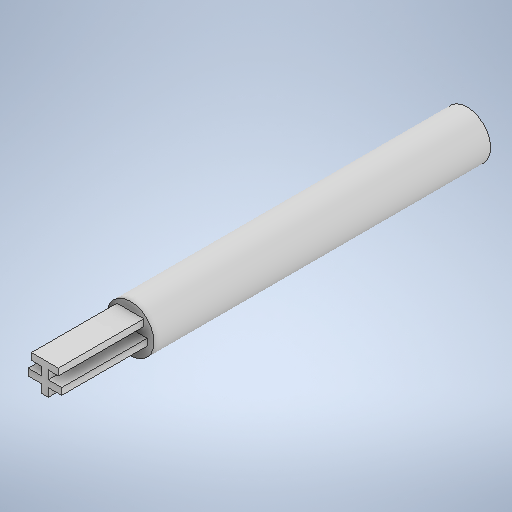
# Autodesk Inventor part: rod attachment(wheelside)
Saved by Autodesk Inventor 2025 (Build 290162000, 162)
## iProperties
Created: 2025-01-07
Part Number: rod attachment(wheelside)
Material: Generic
Document SubType Name: Modeling
Designer: 5014070
Density: 1 g/cm^3
Appearance: Default
Author: 5014070
Autodesk Inventor part; units mm, degrees
ref_plane "YZ Plane" through (0, 0, 0) normal (1, 0, 0) x (0, 1, 0)
ref_plane "XZ Plane" through (0, 0, 0) normal (0, 1, 0) x (-1, 0, 0)
ref_plane "XY Plane" through (0, 0, 0) normal (0, 0, 1) x (1, 0, 0)
sketch "Sketch1" plane through (0, 0, 0) normal (0, 0, 1) x (1, 0, 0)
  circle A0 centre (0, 0) radius 7
  dimension "d0" = 14
  constraints: 1 centre point, 1 coincident
  measures "d0" diameter of A0
extrude "Extrusion1" add sketch "Sketch1" along normal blind 100
sketch "Sketch2" plane through (0, 0, 100) normal (0, 0, 1) x (1, 0, 0)
  line L0 (-1, -4.5) -> (-1, 4.5)
  line L1 (-1, 4.5) -> (1, 4.5)
  line L2 (1, 4.5) -> (1, -4.5)
  line L3 (1, -4.5) -> (-1, -4.5)
  line L4 (-1, -4.5) -> (1, 4.5) construction
  line L5 (-1, 4.5) -> (1, -4.5) construction
  line L6 (0, 4.5) -> (0, 2.5)
  line L7 (0, 2.5) -> (4, 2.5)
  line L8 (4, 2.5) -> (4, 4.5)
  line L9 (4, 4.5) -> (0, 4.5)
  line L10 (0, 4.5) -> (0, 2.5)
  line L11 (0, 2.5) -> (-4, 2.5)
  line L12 (-4, 2.5) -> (-4, 4.5)
  line L13 (-4, 4.5) -> (0, 4.5)
  line L14 (0, 0) -> (0, -2)
  line L15 (0, -2) -> (-5, -2)
  line L16 (-5, -2) -> (-5, 0)
  line L17 (-5, 0) -> (0, 0)
  line L18 (0, -2) -> (0, 0)
  line L19 (0, 0) -> (5, 0)
  line L20 (5, 0) -> (5, -2)
  line L21 (5, -2) -> (0, -2)
  point P0 (1, 2.5)
  point P1 (-1, 2.5)
  point P2 (-1, 0)
  point P3 (-1, -2)
  point P4 (1, -2)
  point P5 (1, 0)
  dimension "d9" = 9
  dimension "d10" = 2
  dimension "d11" = 2
  dimension "d12" = 4
  dimension "d13" = 4
  dimension "d14" = 2
  dimension "d15" = 5
  dimension "d16" = 5
  constraints: 44 end point, 10 parallel, 8 perpendicular, 3 midpoint, 1 point on line, 1 vertical
  measures "d9" distance of L0.start L0.end
  measures "d10" distance of L0.end L1.end
  measures "d11" distance of L6.start L6.end
  measures "d12" distance of L7.end L6.end
  measures "d13" distance of L6.end L11.end
  measures "d14" distance of L14.start L14.end
  measures "d15" distance of L16.end L14.start
  measures "d16" distance of L20.end L14.end
extrude "Extrusion2" add sketch "Sketch2" along normal blind 25.4
sketch "Sketch3" plane through (0, 0, 0) normal (0, 0, -1) x (-1, 0, 0)
  circle A0 centre (0, 0) radius 4
  dimension "d17" = 8
  constraints: 1 centre point, 1 coincident
  measures "d17" diameter of A0
body "Solid1"
